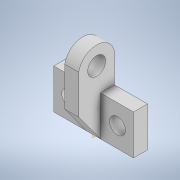
# Autodesk Inventor part: 14
Saved by Autodesk Inventor 2022 (Build 260153000, 153)
## iProperties
Created: 2022-03-14
Part Number: 14
Material: Všeobecné
Document SubType Name: Modeling
Designer: Šimon
Density: 1 g/cm^3
Appearance: Výchozí
Author: Šimon
Autodesk Inventor part; units mm, degrees
ref_plane "XZ Plane" through (0, 0, 0) normal (0, 1, 0) x (-1, 0, 0)
ref_plane "XY Plane" through (0, 0, 0) normal (0, 0, 1) x (1, 0, 0)
sketch "Náčrt1" plane through (0, 0, 0) normal (0, 0, 1) x (1, 0, 0)
  line L0 (0, 0) -> (80, 0)
  line L1 (80, 0) -> (80, 40)
  line L2 (80, 40) -> (0, 40)
  line L3 (0, 40) -> (0, 0)
  circle A0 centre (16, 20) radius 8
  circle A1 centre (64, 20) radius 8
  dimension "d0" = 80
  dimension "d1" = 40
  dimension "d2" = 16
  dimension "d3" = 16
  constraints: 8 end point, 2 centre point, 2 parallel, 1 horizontal, 1 perpendicular
  measures "d0" distance of L2.end L1.end
  measures "d1" distance of L1.end L0.end
  measures "d2" diameter of A0
  measures "d3" diameter of A1
extrude "Vysunutí1" add sketch "Náčrt1" against normal blind 14
ref_plane "Pracovní rovina1" through (40, 0, 0) normal (1, 0, 0) x (0, 1, 0)
sketch "Náčrt2" plane through (40, 0, 0) normal (1, 0, 0) x (0, 1, 0)
  line L0 (0, -14) -> (40, -14) projected
  line L1 (40, -14) -> (69, -14)
  line L2 (40, 0) -> (0, 0) projected
  circle A0 centre (65.4628, 4) radius 9
  arc A1 (69, -14) -> (69, 22) centre (65.4628, 4) ccw
  line L3 (69, 22) -> (30, 22)
  line L4 (30, 22) -> (0, 0)
  line L5 (0, 0) -> (0, -14)
  line L6 (0, -14) -> (40, -14)
  dimension "d7" = 29
  dimension "d9" = 18
  dimension "d10" = 36
  dimension "d11" = 18.3443
  dimension "d12" = 39
  constraints: 10 end point, 2 centre point, 2 horizontal, 2 point on circle, 1 coincident, 1 perpendicular
  measures "d7" distance of L0.end L1.end
  measures "d9" diameter of A0
  measures "d10" distance of L1.end L3.start
  measures "d11" radius of A1
  measures "d12" distance of L3.start L3.end
extrude "Vysunutí2" add sketch "Náčrt2" along normal mid plane 14
